Autodesk Inventor part; units mm, degrees
(part 2 of 2)
  arc A175 (-42.6526, 43.6661) -> (-42.977, 43.2779) centre (-40.6002, 41.6214) ccw
  line L41 (-42.977, 43.2779) -> (-43.1067, 43.0917)
  line L42 (-43.1067, 43.0917) -> (-41.872, 41.9259)
  line L43 (-41.872, 41.9259) -> (-40.6373, 40.7601)
  line L44 (-40.6373, 40.7601) -> (-40.3848, 41.0649)
  arc A176 (-39.3586, 42.1603) -> (-40.3848, 41.0649) centre (-30.9209, 33.2272) ccw
  arc A177 (-38.2304, 43.0935) -> (-39.3586, 42.1603) centre (-31.7148, 34.0677) ccw
  arc A178 (-37.0066, 43.858) -> (-38.2304, 43.0935) centre (-31.9087, 34.3364) ccw
  arc A179 (-35.6955, 44.45) -> (-37.0066, 43.858) centre (-31.97, 34.4509) ccw
  arc A180 (-32.3301, 45.1442) -> (-35.6955, 44.45) centre (-31.7654, 33.9017) ccw
  arc A181 (-28.9479, 44.7788) -> (-32.3301, 45.1442) centre (-31.7871, 34.3342) ccw
  arc A182 (-25.8331, 43.3785) -> (-28.9479, 44.7788) centre (-31.8114, 34.245) ccw
  arc A183 (-23.2452, 41.0656) -> (-25.8331, 43.3785) centre (-32.202, 33.6483) ccw
  line L45 (-23.2452, 41.0656) -> (-22.9934, 40.7615)
  line L46 (-22.9934, 40.7615) -> (-21.7595, 41.928)
  line L47 (-21.7595, 41.928) -> (-20.5256, 43.0945)
  line L48 (-20.5256, 43.0945) -> (-20.6545, 43.2793)
  arc A184 (-20.6545, 43.2793) -> (-20.7446, 43.3915) centre (-21.5367, 42.6637) ccw
  arc A185 (-20.7446, 43.3915) -> (-20.9906, 43.656) centre (-42.9217, 23.0143) ccw
  arc A186 (-20.9906, 43.656) -> (-21.2887, 43.9678) centre (-41.1575, 24.6748) ccw
  arc A187 (-21.2887, 43.9678) -> (-21.6175, 44.3024) centre (-49.0563, 17.0049) ccw
  arc A188 (-21.6175, 44.3024) -> (-22.5505, 45.1704) centre (-33.3143, 32.6659) ccw
  arc A189 (-22.5505, 45.1704) -> (-23.4953, 45.9106) centre (-31.0271, 35.323) ccw
  arc A190 (-23.4953, 45.9106) -> (-24.5028, 46.5592) centre (-31, 35.361) ccw
  arc A191 (-24.5028, 46.5592) -> (-25.6239, 47.1525) centre (-32.6544, 32.5096) ccw
  arc A192 (-25.6239, 47.1525) -> (-26.7379, 47.628) centre (-31.5598, 34.7894) ccw
  arc A193 (-26.7379, 47.628) -> (-27.9121, 48.0141) centre (-31.9655, 33.7091) ccw
  arc A194 (-27.9121, 48.0141) -> (-29.1159, 48.3018) centre (-31.976, 33.6721) ccw
  arc A195 (-29.1159, 48.3018) -> (-30.3185, 48.4827) centre (-31.7827, 34.6607) ccw
  arc A196 (-30.3185, 48.4827) -> (-30.9625, 48.5251) centre (-31.1728, 40.418) ccw
  arc A197 (-30.9625, 48.5251) -> (-31.8952, 48.5365) centre (-31.8434, 14.5791) ccw
  arc A198 (-31.8952, 48.5365) -> (-32.8196, 48.5227) centre (-31.8427, 14.0809) ccw
  arc A199 (-32.8196, 48.5227) -> (-33.4163, 48.478) centre (-32.6367, 42.0762) ccw
  arc A200 (-32.4307, 43.0264) -> (-34.0237, 42.7492) centre (-31.3613, 32.1655) ccw
  arc A201 (-34.0237, 42.7492) -> (-35.4688, 42.2479) centre (-31.8884, 34.261) ccw
  arc A202 (-35.4688, 42.2479) -> (-36.7759, 41.515) centre (-32.0428, 34.6053) ccw
  arc A203 (-36.7759, 41.515) -> (-37.9581, 40.5486) centre (-31.6765, 34.0706) ccw
  arc A204 (-37.9581, 40.5486) -> (-38.3376, 40.1652) centre (-28.7647, 31.0677) ccw
  arc A205 (-38.3376, 40.1652) -> (-38.6996, 39.7682) centre (-28.9248, 31.2199) ccw
  arc A206 (-38.6996, 39.7682) -> (-39.0151, 39.4003) centre (-20.0519, 23.4603) ccw
  arc A207 (-39.0151, 39.4003) -> (-39.0527, 39.2969) centre (-38.8921, 39.2969) ccw
  arc A208 (-39.0527, 39.2969) -> (-39.0335, 39.2524) centre (-38.9916, 39.2969) ccw
  arc A209 (-39.0335, 39.2524) -> (-37.8449, 38.1333) centre (2906.6809, 3166.558) ccw
  arc A210 (-37.8449, 38.1333) -> (-36.672, 37.0301) centre (1469.8323, 1639.9712) ccw
  arc A211 (-36.672, 37.0301) -> (-36.5889, 36.978) centre (-36.4978, 37.2154) ccw
  arc A212 (-36.5889, 36.978) -> (-36.5603, 36.9845) centre (-36.5795, 37.0026) ccw
  arc A213 (-36.5603, 36.9845) -> (-36.4741, 37.0791) centre (-39.0948, 39.3809) ccw
  arc A214 (-36.4741, 37.0791) -> (-36.3741, 37.2003) centre (-38.4073, 38.777) ccw
  arc A215 (-36.3741, 37.2003) -> (-36.2643, 37.3476) centre (-40.1553, 40.1326) ccw
  arc A216 (-35.6055, 38.1053) -> (-36.2643, 37.3476) centre (-31.9353, 34.249) ccw
  arc A217 (-34.8086, 38.7361) -> (-35.6055, 38.1053) centre (-31.7546, 34.0592) ccw
  arc A218 (-33.9056, 39.2153) -> (-34.8086, 38.7361) centre (-31.7182, 34.0034) ccw
  arc A219 (-32.9322, 39.5234) -> (-33.9056, 39.2153) centre (-31.7286, 34.0282) ccw
  arc A220 (-32.3612, 39.5988) -> (-32.9322, 39.5234) centre (-32.201, 36.1851) ccw
  arc A221 (-31.6217, 39.6035) -> (-32.3612, 39.5988) centre (-31.9333, 30.4803) ccw
  arc A222 (-30.8835, 39.5483) -> (-31.6217, 39.6035) centre (-31.9336, 30.4734) ccw
  arc A223 (-30.3166, 39.434) -> (-30.8835, 39.5483) centre (-31.2817, 36.1076) ccw
  arc A224 (-29.4512, 39.0947) -> (-30.3166, 39.434) centre (-31.7361, 34.5412) ccw
  arc A225 (-28.6193, 38.5905) -> (-29.4512, 39.0947) centre (-32.1874, 33.6419) ccw
  arc A226 (-27.8809, 37.9625) -> (-28.6193, 38.5905) centre (-32.1638, 33.6746) ccw
  arc A227 (-27.2937, 37.2545) -> (-27.8809, 37.9625) centre (-31.3579, 34.4814) ccw
  arc A228 (-27.2937, 37.2545) -> (-27.2128, 37.1424) centre (-25.1615, 38.7093) ccw
  arc A229 (-27.2128, 37.1424) -> (-27.1366, 37.051) centre (-26.0837, 38.0049) ccw
  arc A230 (-27.1366, 37.051) -> (-27.071, 36.9831) centre (-26.0649, 38.0219) ccw
  arc A231 (-27.071, 36.9831) -> (-27.0426, 36.9773) centre (-27.0522, 37.0025) ccw
  arc A232 (-27.0426, 36.9773) -> (-26.9623, 37.0275) centre (-27.13, 37.2061) ccw
  arc A233 (-26.9623, 37.0275) -> (-25.7864, 38.1315) centre (-1649.919, 1766.8952) ccw
  arc A234 (-25.7864, 38.1315) -> (-24.5953, 39.2509) centre (-3169.5689, 3384.4472) ccw
  arc A235 (-24.5953, 39.2509) -> (-24.5767, 39.2939) centre (-24.6358, 39.2939) ccw
  arc A236 (-24.5767, 39.2939) -> (-24.5825, 39.3115) centre (-24.6064, 39.2939) ccw
  arc A237 (-24.5825, 39.3115) -> (-24.6669, 39.4252) centre (-44.5732, 24.5671) ccw
  arc A238 (-24.6669, 39.4252) -> (-24.766, 39.5554) centre (-31.6067, 34.2453) ccw
  arc A239 (-24.766, 39.5554) -> (-24.8836, 39.7051) centre (-37.2564, 29.8598) ccw
  arc A240 (-24.8836, 39.7051) -> (-25.4949, 40.3815) centre (-30.5776, 35.1743) ccw
  arc A241 (-25.4949, 40.3815) -> (-26.2501, 41.0537) centre (-33.1647, 32.5237) ccw
  arc A242 (-26.2501, 41.0537) -> (-27.0662, 41.6552) centre (-33.1968, 32.4842) ccw
  arc A243 (-27.0662, 41.6552) -> (-27.8611, 42.1187) centre (-31.2352, 35.4187) ccw
  arc A244 (-27.8611, 42.1187) -> (-28.3727, 42.3447) centre (-30.3506, 37.1753) ccw
  arc A245 (-28.3727, 42.3447) -> (-29.0377, 42.5799) centre (-33.3146, 29.4285) ccw
  arc A246 (-29.0377, 42.5799) -> (-29.717, 42.7818) centre (-33.3337, 29.3697) ccw
  arc A247 (-29.717, 42.7818) -> (-30.2747, 42.9036) centre (-31.2556, 37.0763) ccw
  arc A248 (-30.2747, 42.9036) -> (-30.7758, 42.9692) centre (-31.4176, 36.1138) ccw
  arc A249 (-30.7758, 42.9692) -> (-31.4147, 43.0173) centre (-32.4141, 25.4701) ccw
  arc A250 (-31.4147, 43.0173) -> (-32.0314, 43.0416) centre (-32.4232, 25.3115) ccw
  arc A251 (-32.0314, 43.0416) -> (-32.4307, 43.0264) centre (-32.1049, 39.7171) ccw
  arc A252 (-32.5231, 37.4314) -> (-33.3556, 37.0457) centre (-31.7598, 34.6924) ccw
  arc A253 (-33.3556, 37.0457) -> (-34.029, 36.4127) centre (-31.7134, 34.624) ccw
  arc A254 (-34.029, 36.4127) -> (-34.4667, 35.6071) centre (-31.7526, 34.6543) ccw
  arc A255 (-34.4667, 35.6071) -> (-34.6168, 34.7211) centre (-31.9577, 34.7263) ccw
  arc A256 (-34.6168, 34.7211) -> (-34.3295, 33.4989) centre (-31.8505, 34.7265) ccw
  arc A257 (-34.3295, 33.4989) -> (-33.5302, 32.5168) centre (-31.7681, 34.7673) ccw
  arc A258 (-33.5302, 32.5168) -> (-32.39, 31.9809) centre (-31.7888, 34.7408) ccw
  arc A259 (-32.39, 31.9809) -> (-31.149, 32.0059) centre (-31.8219, 34.5891) ccw
  arc A260 (-31.149, 32.0059) -> (-30.4318, 32.2925) centre (-31.9281, 34.9968) ccw
  arc A261 (-30.4318, 32.2925) -> (-29.8377, 32.7398) centre (-31.7217, 34.6238) ccw
  arc A262 (-29.8377, 32.7398) -> (-29.3904, 33.3339) centre (-31.7217, 34.6238) ccw
  arc A263 (-29.3904, 33.3339) -> (-29.1038, 34.0512) centre (-32.0947, 34.8302) ccw
  arc A264 (-29.1038, 34.0512) -> (-29.0802, 35.3061) centre (-31.7012, 34.7277) ccw
  arc A265 (-29.0802, 35.3061) -> (-29.6276, 36.4511) centre (-31.8129, 34.703) ccw
  arc A266 (-29.6276, 36.4511) -> (-30.6294, 37.2438) centre (-31.8465, 34.6762) ccw
  arc A267 (-30.6294, 37.2438) -> (-31.8739, 37.5142) centre (-31.8323, 34.7062) ccw
  arc A268 (-31.8739, 37.5142) -> (-32.0366, 37.5064) centre (-31.837, 35.023) ccw
  arc A269 (-32.0366, 37.5064) -> (-32.2181, 37.4876) centre (-31.7229, 33.6029) ccw
  arc A270 (-32.2181, 37.4876) -> (-32.3905, 37.4614) centre (-31.75, 33.8157) ccw
  arc A271 (-32.3905, 37.4614) -> (-32.5231, 37.4314) centre (-32.15, 36.0926) ccw
  arc A272 (-54.2587, 71.8195) -> (-55.2164, 71.6633) centre (-53.721, 65.5053) ccw
  arc A273 (-55.2164, 71.6633) -> (-56.1281, 71.3638) centre (-53.7854, 65.7705) ccw
  arc A274 (-56.1281, 71.3638) -> (-56.9803, 70.9245) centre (-53.7898, 65.7811) ccw
  arc A275 (-56.9803, 70.9245) -> (-57.761, 70.3525) centre (-53.6689, 65.5862) ccw
  arc A276 (-57.761, 70.3525) -> (-57.9303, 70.1998) centre (-54.7143, 66.8038) ccw
  arc A277 (-57.9303, 70.1998) -> (-58.1244, 70.0106) centre (-51.5447, 63.4568) ccw
  arc A278 (-58.1244, 70.0106) -> (-58.3037, 69.8254) centre (-51.7023, 63.6139) ccw
  arc A279 (-58.3037, 69.8254) -> (-58.4189, 69.6921) centre (-56.7958, 68.4066) ccw
  line L49 (-58.4189, 69.6921) -> (-58.4764, 69.6194)
  line L50 (-58.4764, 69.6194) -> (-58.0951, 69.2684)
  line L51 (-58.0951, 69.2684) -> (-57.7138, 68.9174)
  line L52 (-57.7138, 68.9174) -> (-57.6118, 69.0338)
  arc A280 (-57.0139, 69.616) -> (-57.6118, 69.0338) centre (-53.6679, 65.5813) ccw
  arc A281 (-56.3308, 70.0963) -> (-57.0139, 69.616) centre (-53.6618, 65.5739) ccw
  arc A282 (-55.5869, 70.4582) -> (-56.3308, 70.0963) centre (-53.7111, 65.6576) ccw
  arc A283 (-54.8079, 70.6887) -> (-55.5869, 70.4582) centre (-53.8421, 65.9928) ccw
  arc A284 (-54.2943, 70.7669) -> (-54.8079, 70.6887) centre (-53.7974, 65.7752) ccw
  arc A285 (-53.7678, 70.793) -> (-54.2943, 70.7669) centre (-53.7678, 65.4777) ccw
  arc A286 (-53.2413, 70.7669) -> (-53.7678, 70.793) centre (-53.7678, 65.4777) ccw
  arc A287 (-52.7277, 70.6887) -> (-53.2413, 70.7669) centre (-53.7382, 65.7752) ccw
  arc A288 (-51.9486, 70.4585) -> (-52.7277, 70.6887) centre (-53.6976, 65.9726) ccw
  arc A289 (-51.2067, 70.0979) -> (-51.9486, 70.4585) centre (-53.8074, 65.6909) ccw
  arc A290 (-50.5247, 69.6182) -> (-51.2067, 70.0979) centre (-53.8645, 65.5942) ccw
  arc A291 (-49.9239, 69.034) -> (-50.5247, 69.6182) centre (-53.9323, 65.5125) ccw
  line L53 (-49.9239, 69.034) -> (-49.8218, 68.9178)
  line L54 (-49.8218, 68.9178) -> (-49.4403, 69.2684)
  line L55 (-49.4403, 69.2684) -> (-49.0588, 69.619)
  line L56 (-49.0588, 69.619) -> (-49.1187, 69.6961)
  arc A292 (-49.1187, 69.6961) -> (-49.2435, 69.8387) centre (-50.3783, 68.7188) ccw
  arc A293 (-49.2435, 69.8387) -> (-49.4908, 70.0838) centre (-60.4502, 58.7794) ccw
  arc A294 (-49.4908, 70.0838) -> (-49.7488, 70.3278) centre (-59.4752, 59.7852) ccw
  arc A295 (-49.7488, 70.3278) -> (-49.9351, 70.4876) centre (-52.0641, 67.8182) ccw
  arc A296 (-49.9351, 70.4876) -> (-50.698, 71.0097) centre (-53.8793, 65.5422) ccw
  arc A297 (-50.698, 71.0097) -> (-51.5212, 71.4089) centre (-53.7491, 65.766) ccw
  arc A298 (-51.5212, 71.4089) -> (-52.3959, 71.6801) centre (-53.7544, 65.7527) ccw
  arc A299 (-52.3959, 71.6801) -> (-53.3127, 71.8212) centre (-53.8245, 65.4466) ccw
  arc A300 (-53.3127, 71.8212) -> (-53.5357, 71.8337) centre (-53.6841, 67.195) ccw
  arc A301 (-53.5357, 71.8337) -> (-53.7872, 71.8375) centre (-53.7737, 64.3958) ccw
  arc A302 (-53.7872, 71.8375) -> (-54.0379, 71.8328) centre (-53.7737, 64.4287) ccw
  arc A303 (-54.0379, 71.8328) -> (-54.2587, 71.8195) centre (-53.8779, 67.3479) ccw
  arc A304 (-54.2587, 70.1206) -> (-54.8466, 70.011) centre (-53.685, 65.4098) ccw
  arc A305 (-54.8466, 70.011) -> (-55.4044, 69.8298) centre (-53.7721, 65.755) ccw
  arc A306 (-55.4044, 69.8298) -> (-55.9344, 69.5753) centre (-53.7639, 65.7344) ccw
  arc A307 (-55.9344, 69.5753) -> (-56.4394, 69.2471) centre (-53.5452, 65.3475) ccw
  arc A308 (-56.4394, 69.2471) -> (-56.6021, 69.1131) centre (-55.1906, 67.5645) ccw
  arc A309 (-56.6021, 69.1131) -> (-56.8494, 68.8817) centre (-47.9272, 59.5958) ccw
  arc A310 (-56.8494, 68.8817) -> (-57.0896, 68.6458) centre (-46.1793, 57.7765) ccw
  arc A311 (-57.0896, 68.6458) -> (-57.189, 68.5268) centre (-56.4605, 68.0191) ccw
  line L57 (-57.189, 68.5268) -> (-57.2288, 68.4697)
  line L58 (-57.2288, 68.4697) -> (-56.8503, 68.1124)
  line L59 (-56.8503, 68.1124) -> (-56.4719, 67.7551)
  line L60 (-56.4719, 67.7551) -> (-56.3945, 67.8485)
  arc A312 (-56.08, 68.1842) -> (-56.3945, 67.8485) centre (-53.4938, 65.4462) ccw
  arc A313 (-55.7342, 68.4703) -> (-56.08, 68.1842) centre (-53.7371, 65.7039) ccw
  arc A314 (-55.3591, 68.7046) -> (-55.7342, 68.4703) centre (-53.7966, 65.7862) ccw
  arc A315 (-54.9572, 68.886) -> (-55.3591, 68.7046) centre (-53.8154, 65.8213) ccw
  arc A316 (-53.9257, 69.0988) -> (-54.9572, 68.886) centre (-53.7527, 65.653) ccw
  arc A317 (-52.8891, 68.9868) -> (-53.9257, 69.0988) centre (-53.7593, 65.7856) ccw
  arc A318 (-51.9344, 68.5576) -> (-52.8891, 68.9868) centre (-53.7667, 65.7582) ccw
  arc A319 (-51.1412, 67.8487) -> (-51.9344, 68.5576) centre (-53.8865, 65.5753) ccw
  line L61 (-51.1412, 67.8487) -> (-51.064, 67.7555)
  line L62 (-51.064, 67.7555) -> (-50.6858, 68.113)
  line L63 (-50.6858, 68.113) -> (-50.3077, 68.4706)
  line L64 (-50.3077, 68.4706) -> (-50.3472, 68.5272)
  arc A320 (-50.3472, 68.5272) -> (-50.3748, 68.5616) centre (-50.6176, 68.3385) ccw
  arc A321 (-50.3748, 68.5616) -> (-50.4502, 68.6427) centre (-57.1721, 62.316) ccw
  arc A322 (-50.4502, 68.6427) -> (-50.5416, 68.7383) centre (-56.6313, 62.825) ccw
  arc A323 (-50.5416, 68.7383) -> (-50.6423, 68.8408) centre (-59.0523, 60.4741) ccw
  arc A324 (-50.6423, 68.8408) -> (-50.9283, 69.1069) centre (-54.2274, 65.2742) ccw
  arc A325 (-50.9283, 69.1069) -> (-51.2179, 69.3337) centre (-53.5264, 66.0886) ccw
  arc A326 (-51.2179, 69.3337) -> (-51.5267, 69.5325) centre (-53.5181, 66.1003) ccw
  arc A327 (-51.5267, 69.5325) -> (-51.8703, 69.7143) centre (-54.0251, 65.2263) ccw
  arc A328 (-51.8703, 69.7143) -> (-52.2117, 69.8601) centre (-53.6897, 65.9251) ccw
  arc A329 (-52.2117, 69.8601) -> (-52.5716, 69.9784) centre (-53.814, 65.594) ccw
  arc A330 (-52.5716, 69.9784) -> (-52.9406, 70.0666) centre (-53.8172, 65.5826) ccw
  arc A331 (-52.9406, 70.0666) -> (-53.3092, 70.1221) centre (-53.758, 65.8856) ccw
  arc A332 (-53.3092, 70.1221) -> (-53.5066, 70.1351) centre (-53.571, 67.6502) ccw
  arc A333 (-53.5066, 70.1351) -> (-53.7925, 70.1386) centre (-53.7766, 59.7306) ccw
  arc A334 (-53.7925, 70.1386) -> (-54.0758, 70.1343) centre (-53.7763, 59.5779) ccw
  arc A335 (-54.0758, 70.1343) -> (-54.2587, 70.1206) centre (-54.0197, 68.1585) ccw
  arc A336 (-53.9566, 68.4497) -> (-54.4448, 68.3648) centre (-53.6288, 65.1208) ccw
  arc A337 (-54.4448, 68.3648) -> (-54.8878, 68.2111) centre (-53.7904, 65.7631) ccw
  arc A338 (-54.8878, 68.2111) -> (-55.2884, 67.9865) centre (-53.8377, 65.8687) ccw
  arc A339 (-55.2884, 67.9865) -> (-55.6507, 67.6903) centre (-53.7254, 65.7048) ccw
  arc A340 (-55.6507, 67.6903) -> (-55.7671, 67.5728) centre (-52.8329, 64.7844) ccw
  arc A341 (-55.7671, 67.5728) -> (-55.878, 67.4511) centre (-52.882, 64.831) ccw
  arc A342 (-55.878, 67.4511) -> (-55.9747, 67.3383) centre (-50.1625, 62.4527) ccw
  arc A343 (-55.9747, 67.3383) -> (-55.9862, 67.3066) centre (-55.937, 67.3066) ccw
  arc A344 (-55.9862, 67.3066) -> (-55.9803, 67.293) centre (-55.9675, 67.3066) ccw
  arc A345 (-55.9803, 67.293) -> (-55.616, 66.95) centre (846.8811, 1025.8121) ccw
  arc A346 (-55.616, 66.95) -> (-55.2565, 66.6118) centre (406.487, 557.9133) ccw
  arc A347 (-55.2565, 66.6118) -> (-55.2311, 66.5959) centre (-55.2031, 66.6687) ccw
  arc A348 (-55.2311, 66.5959) -> (-55.2223, 66.5979) centre (-55.2282, 66.6034) ccw
  arc A349 (-55.2223, 66.5979) -> (-55.1959, 66.6269) centre (-55.9991, 67.3324) ccw
  arc A350 (-55.1959, 66.6269) -> (-55.1652, 66.664) centre (-55.7884, 67.1473) ccw
  arc A351 (-55.1652, 66.664) -> (-55.1316, 66.7092) centre (-56.3242, 67.5628) ccw
  arc A352 (-54.9296, 66.9414) -> (-55.1316, 66.7092) centre (-53.8047, 65.7595) ccw
  arc A353 (-54.6854, 67.1347) -> (-54.9296, 66.9414) centre (-53.7494, 65.7013) ccw
  arc A354 (-54.4086, 67.2816) -> (-54.6854, 67.1347) centre (-53.7382, 65.6842) ccw
  arc A355 (-54.1103, 67.376) -> (-54.4086, 67.2816) centre (-53.7414, 65.6918) ccw
  arc A356 (-53.9353, 67.3991) -> (-54.1103, 67.376) centre (-53.8862, 66.3529) ccw
  arc A357 (-53.7086, 67.4006) -> (-53.9353, 67.3991) centre (-53.8041, 64.6043) ccw
  arc A358 (-53.4824, 67.3837) -> (-53.7086, 67.4006) centre (-53.8042, 64.6022) ccw
  arc A359 (-53.3086, 67.3487) -> (-53.4824, 67.3837) centre (-53.6044, 66.3291) ccw
  arc A360 (-53.0433, 67.2446) -> (-53.3086, 67.3487) centre (-53.7437, 65.849) ccw
  arc A361 (-52.7884, 67.0901) -> (-53.0433, 67.2446) centre (-53.882, 65.5734) ccw
  arc A362 (-52.562, 66.8976) -> (-52.7884, 67.0901) centre (-53.8748, 65.5834) ccw
  arc A363 (-52.3821, 66.6806) -> (-52.562, 66.8976) centre (-53.6278, 65.8307) ccw
  arc A364 (-52.3821, 66.6806) -> (-52.3573, 66.6463) centre (-51.7286, 67.1265) ccw
  arc A365 (-52.3573, 66.6463) -> (-52.3339, 66.6182) centre (-52.0112, 66.9106) ccw
  arc A366 (-52.3339, 66.6182) -> (-52.3138, 66.5974) centre (-52.0055, 66.9158) ccw
  arc A367 (-52.3138, 66.5974) -> (-52.3051, 66.5957) centre (-52.3081, 66.6034) ccw
  arc A368 (-52.3051, 66.5957) -> (-52.2805, 66.611) centre (-52.3319, 66.6658) ccw
  arc A369 (-52.2805, 66.611) -> (-51.9201, 66.9494) centre (-549.7167, 596.8155) ccw
  arc A370 (-51.9201, 66.9494) -> (-51.555, 67.2925) centre (-1015.4894, 1092.5952) ccw
  arc A371 (-51.555, 67.2925) -> (-51.5493, 67.3057) centre (-51.5674, 67.3057) ccw
  arc A372 (-51.5493, 67.3057) -> (-51.5511, 67.3111) centre (-51.5584, 67.3057) ccw
  arc A373 (-51.5511, 67.3111) -> (-51.577, 67.3459) centre (-57.6783, 62.7919) ccw
  arc A374 (-51.577, 67.3459) -> (-51.6073, 67.3859) centre (-53.704, 65.7583) ccw
  arc A375 (-51.6073, 67.3859) -> (-51.6434, 67.4317) centre (-55.4356, 64.4141) ccw
  arc A376 (-51.6434, 67.4317) -> (-51.8307, 67.6391) centre (-53.3886, 66.043) ccw
  arc A377 (-51.8307, 67.6391) -> (-52.0622, 67.8451) centre (-54.1816, 65.2306) ccw
  arc A378 (-52.0622, 67.8451) -> (-52.3124, 68.0294) centre (-54.1914, 65.2185) ccw
  arc A379 (-52.3124, 68.0294) -> (-52.556, 68.1715) centre (-53.5902, 66.1179) ccw
  arc A380 (-52.556, 68.1715) -> (-52.7128, 68.2408) centre (-53.319, 66.6563) ccw
  arc A381 (-52.7128, 68.2408) -> (-52.9166, 68.3129) centre (-54.2275, 64.282) ccw
  arc A382 (-52.9166, 68.3129) -> (-53.1248, 68.3747) centre (-54.2334, 64.2639) ccw
  arc A383 (-53.1248, 68.3747) -> (-53.2958, 68.4121) centre (-53.5964, 66.626) ccw
  arc A384 (-53.2958, 68.4121) -> (-53.4493, 68.4322) centre (-53.6461, 66.331) ccw
  arc A385 (-53.4493, 68.4322) -> (-53.6452, 68.4469) centre (-53.9515, 63.0687) ccw
  arc A386 (-53.6452, 68.4469) -> (-53.8342, 68.4544) centre (-53.9543, 63.0201) ccw
  arc A387 (-53.8342, 68.4544) -> (-53.9566, 68.4497) centre (-53.8567, 67.4354) ccw
  arc A388 (-53.9849, 66.7348) -> (-54.24, 66.6166) centre (-53.7509, 65.8954) ccw
  arc A389 (-54.24, 66.6166) -> (-54.4464, 66.4226) centre (-53.7367, 65.8744) ccw
  arc A390 (-54.4464, 66.4226) -> (-54.5806, 66.1757) centre (-53.7487, 65.8837) ccw
  arc A391 (-54.5806, 66.1757) -> (-54.6266, 65.9041) centre (-53.8116, 65.9057) ccw
  arc A392 (-54.6266, 65.9041) -> (-54.5386, 65.5295) centre (-53.7788, 65.9058) ccw
  arc A393 (-54.5386, 65.5295) -> (-54.2936, 65.2285) centre (-53.7535, 65.9183) ccw
  arc A394 (-54.2936, 65.2285) -> (-53.9441, 65.0643) centre (-53.7598, 65.9102) ccw
  arc A395 (-53.9441, 65.0643) -> (-53.5637, 65.0719) centre (-53.77, 65.8637) ccw
  arc A396 (-53.5637, 65.0719) -> (-53.3439, 65.1598) centre (-53.8025, 65.9887) ccw
  arc A397 (-53.3439, 65.1598) -> (-53.1618, 65.2969) centre (-53.7393, 65.8743) ccw
  arc A398 (-53.1618, 65.2969) -> (-53.0247, 65.479) centre (-53.7393, 65.8743) ccw
  arc A399 (-53.0247, 65.479) -> (-52.9369, 65.6988) centre (-53.8536, 65.9376) ccw
  arc A400 (-52.9369, 65.6988) -> (-52.9297, 66.0834) centre (-53.733, 65.9062) ccw
  arc A401 (-52.9297, 66.0834) -> (-53.0974, 66.4344) centre (-53.7672, 65.8986) ccw
  arc A402 (-53.0974, 66.4344) -> (-53.4045, 66.6773) centre (-53.7775, 65.8904) ccw
  arc A403 (-53.4045, 66.6773) -> (-53.7859, 66.7602) centre (-53.7732, 65.8996) ccw
  arc A404 (-53.7859, 66.7602) -> (-53.8358, 66.7578) centre (-53.7746, 65.9967) ccw
  arc A405 (-53.8358, 66.7578) -> (-53.8914, 66.7521) centre (-53.7396, 65.5614) ccw
  arc A406 (-53.8914, 66.7521) -> (-53.9443, 66.7441) centre (-53.7479, 65.6266) ccw
  arc A407 (-53.9443, 66.7441) -> (-53.9849, 66.7348) centre (-53.8705, 66.3245) ccw
  arc A408 (-9.2413, 17.0805) -> (-8.2836, 17.2367) centre (-9.779, 23.3947) ccw
  arc A409 (-8.2836, 17.2367) -> (-7.3719, 17.5362) centre (-9.7146, 23.1295) ccw
  arc A410 (-7.3719, 17.5362) -> (-6.5197, 17.9755) centre (-9.7102, 23.1189) ccw
  arc A411 (-6.5197, 17.9755) -> (-5.739, 18.5475) centre (-9.8311, 23.3138) ccw
  arc A412 (-5.739, 18.5475) -> (-5.5697, 18.7002) centre (-8.7857, 22.0962) ccw
  arc A413 (-5.5697, 18.7002) -> (-5.3756, 18.8894) centre (-11.9553, 25.4432) ccw
  arc A414 (-5.3756, 18.8894) -> (-5.1963, 19.0746) centre (-11.7977, 25.2861) ccw
  arc A415 (-5.1963, 19.0746) -> (-5.0811, 19.2079) centre (-6.7042, 20.4934) ccw
  line L65 (-5.0811, 19.2079) -> (-5.0236, 19.2806)
  line L66 (-5.0236, 19.2806) -> (-5.4049, 19.6316)
  line L67 (-5.4049, 19.6316) -> (-5.7862, 19.9826)
  line L68 (-5.7862, 19.9826) -> (-5.8882, 19.8662)
  arc A416 (-6.4861, 19.284) -> (-5.8882, 19.8662) centre (-9.8321, 23.3187) ccw
  arc A417 (-7.1692, 18.8037) -> (-6.4861, 19.284) centre (-9.8382, 23.3261) ccw
  arc A418 (-7.9131, 18.4418) -> (-7.1692, 18.8037) centre (-9.7889, 23.2424) ccw
  arc A419 (-8.6921, 18.2113) -> (-7.9131, 18.4418) centre (-9.6579, 22.9072) ccw
  arc A420 (-9.2057, 18.1331) -> (-8.6921, 18.2113) centre (-9.7026, 23.1248) ccw
  arc A421 (-9.7322, 18.107) -> (-9.2057, 18.1331) centre (-9.7322, 23.4223) ccw
  arc A422 (-10.2587, 18.1331) -> (-9.7322, 18.107) centre (-9.7322, 23.4223) ccw
  arc A423 (-10.7723, 18.2113) -> (-10.2587, 18.1331) centre (-9.7618, 23.1248) ccw
  arc A424 (-11.5514, 18.4415) -> (-10.7723, 18.2113) centre (-9.8024, 22.9274) ccw
  arc A425 (-12.2933, 18.8021) -> (-11.5514, 18.4415) centre (-9.6926, 23.2091) ccw
  arc A426 (-12.9753, 19.2818) -> (-12.2933, 18.8021) centre (-9.6355, 23.3058) ccw
  arc A427 (-13.5761, 19.866) -> (-12.9753, 19.2818) centre (-9.5677, 23.3875) ccw
  line L69 (-13.5761, 19.866) -> (-13.6782, 19.9822)
  line L70 (-13.6782, 19.9822) -> (-14.0597, 19.6316)
  line L71 (-14.0597, 19.6316) -> (-14.4412, 19.281)
  line L72 (-14.4412, 19.281) -> (-14.3813, 19.2039)
  arc A428 (-14.3813, 19.2039) -> (-14.2565, 19.0613) centre (-13.1217, 20.1812) ccw
  arc A429 (-14.2565, 19.0613) -> (-14.0092, 18.8162) centre (-3.0498, 30.1206) ccw
  arc A430 (-14.0092, 18.8162) -> (-13.7512, 18.5722) centre (-4.0248, 29.1148) ccw
  arc A431 (-13.7512, 18.5722) -> (-13.5649, 18.4124) centre (-11.4359, 21.0818) ccw
  arc A432 (-13.5649, 18.4124) -> (-12.802, 17.8903) centre (-9.6207, 23.3578) ccw
  arc A433 (-12.802, 17.8903) -> (-11.9788, 17.4911) centre (-9.7509, 23.134) ccw
  arc A434 (-11.9788, 17.4911) -> (-11.1041, 17.2199) centre (-9.7456, 23.1473) ccw
  arc A435 (-11.1041, 17.2199) -> (-10.1873, 17.0788) centre (-9.6755, 23.4534) ccw
  arc A436 (-10.1873, 17.0788) -> (-9.9643, 17.0663) centre (-9.8159, 21.705) ccw
  arc A437 (-9.9643, 17.0663) -> (-9.7128, 17.0625) centre (-9.7263, 24.5042) ccw
  arc A438 (-9.7128, 17.0625) -> (-9.4621, 17.0672) centre (-9.7263, 24.4713) ccw
  arc A439 (-9.4621, 17.0672) -> (-9.2413, 17.0805) centre (-9.6221, 21.5521) ccw
  arc A440 (-9.2413, 18.7794) -> (-8.6534, 18.889) centre (-9.815, 23.4902) ccw
  arc A441 (-8.6534, 18.889) -> (-8.0956, 19.0702) centre (-9.7279, 23.145) ccw
  arc A442 (-8.0956, 19.0702) -> (-7.5656, 19.3247) centre (-9.7361, 23.1656) ccw
  arc A443 (-7.5656, 19.3247) -> (-7.0606, 19.6529) centre (-9.9548, 23.5525) ccw
  arc A444 (-7.0606, 19.6529) -> (-6.8979, 19.7869) centre (-8.3094, 21.3355) ccw
  arc A445 (-6.8979, 19.7869) -> (-6.6506, 20.0183) centre (-15.5728, 29.3042) ccw
  arc A446 (-6.6506, 20.0183) -> (-6.4104, 20.2542) centre (-17.3207, 31.1235) ccw
  arc A447 (-6.4104, 20.2542) -> (-6.311, 20.3732) centre (-7.0395, 20.8809) ccw
  line L73 (-6.311, 20.3732) -> (-6.2712, 20.4303)
  line L74 (-6.2712, 20.4303) -> (-6.6497, 20.7876)
  line L75 (-6.6497, 20.7876) -> (-7.0281, 21.1449)
  line L76 (-7.0281, 21.1449) -> (-7.1055, 21.0515)
  arc A448 (-7.42, 20.7158) -> (-7.1055, 21.0515) centre (-10.0062, 23.4538) ccw
  arc A449 (-7.7658, 20.4297) -> (-7.42, 20.7158) centre (-9.7629, 23.1961) ccw
  arc A450 (-8.1409, 20.1954) -> (-7.7658, 20.4297) centre (-9.7034, 23.1138) ccw
  arc A451 (-8.5428, 20.014) -> (-8.1409, 20.1954) centre (-9.6846, 23.0787) ccw
  arc A452 (-9.5743, 19.8012) -> (-8.5428, 20.014) centre (-9.7473, 23.247) ccw
  arc A453 (-10.6109, 19.9132) -> (-9.5743, 19.8012) centre (-9.7407, 23.1144) ccw
  arc A454 (-11.5656, 20.3424) -> (-10.6109, 19.9132) centre (-9.7333, 23.1418) ccw
  arc A455 (-12.3588, 21.0513) -> (-11.5656, 20.3424) centre (-9.6135, 23.3247) ccw
  line L77 (-12.3588, 21.0513) -> (-12.436, 21.1445)
  line L78 (-12.436, 21.1445) -> (-12.8142, 20.787)
  line L79 (-12.8142, 20.787) -> (-13.1923, 20.4294)
  line L80 (-13.1923, 20.4294) -> (-13.1528, 20.3728)
  arc A456 (-13.1528, 20.3728) -> (-13.1252, 20.3384) centre (-12.8824, 20.5615) ccw
  arc A457 (-13.1252, 20.3384) -> (-13.0498, 20.2573) centre (-6.3279, 26.584) ccw
  arc A458 (-13.0498, 20.2573) -> (-12.9584, 20.1617) centre (-6.8687, 26.075) ccw
  arc A459 (-12.9584, 20.1617) -> (-12.8577, 20.0592) centre (-4.4477, 28.4259) ccw
  arc A460 (-12.8577, 20.0592) -> (-12.5717, 19.7931) centre (-9.2726, 23.6258) ccw
  arc A461 (-12.5717, 19.7931) -> (-12.2821, 19.5663) centre (-9.9736, 22.8114) ccw
  arc A462 (-12.2821, 19.5663) -> (-11.9733, 19.3675) centre (-9.9819, 22.7997) ccw
  arc A463 (-11.9733, 19.3675) -> (-11.6297, 19.1857) centre (-9.4749, 23.6737) ccw
  arc A464 (-11.6297, 19.1857) -> (-11.2883, 19.0399) centre (-9.8103, 22.9749) ccw
  arc A465 (-11.2883, 19.0399) -> (-10.9284, 18.9216) centre (-9.686, 23.306) ccw
  arc A466 (-10.9284, 18.9216) -> (-10.5594, 18.8334) centre (-9.6828, 23.3174) ccw
  arc A467 (-10.5594, 18.8334) -> (-10.1908, 18.7779) centre (-9.742, 23.0144) ccw
  arc A468 (-10.1908, 18.7779) -> (-9.9934, 18.7649) centre (-9.929, 21.2498) ccw
  arc A469 (-9.9934, 18.7649) -> (-9.7075, 18.7614) centre (-9.7234, 29.1694) ccw
  arc A470 (-9.7075, 18.7614) -> (-9.4242, 18.7657) centre (-9.7237, 29.3221) ccw
  arc A471 (-9.4242, 18.7657) -> (-9.2413, 18.7794) centre (-9.4803, 20.7415) ccw
  arc A472 (-9.5434, 20.4503) -> (-9.0552, 20.5352) centre (-9.8712, 23.7792) ccw
  arc A473 (-9.0552, 20.5352) -> (-8.6122, 20.6889) centre (-9.7096, 23.1369) ccw
  arc A474 (-8.6122, 20.6889) -> (-8.2116, 20.9135) centre (-9.6623, 23.0313) ccw
  arc A475 (-8.2116, 20.9135) -> (-7.8493, 21.2097) centre (-9.7746, 23.1952) ccw
  arc A476 (-7.8493, 21.2097) -> (-7.7329, 21.3272) centre (-10.6671, 24.1156) ccw
  arc A477 (-7.7329, 21.3272) -> (-7.622, 21.4489) centre (-10.618, 24.069) ccw
  arc A478 (-7.622, 21.4489) -> (-7.5253, 21.5617) centre (-13.3375, 26.4473) ccw
  arc A479 (-7.5253, 21.5617) -> (-7.5138, 21.5934) centre (-7.563, 21.5934) ccw
  arc A480 (-7.5138, 21.5934) -> (-7.5197, 21.607) centre (-7.5325, 21.5934) ccw
  arc A481 (-7.5197, 21.607) -> (-7.884, 21.95) centre (-910.3811, -936.9121) ccw
  arc A482 (-7.884, 21.95) -> (-8.2435, 22.2882) centre (-469.987, -469.0133) ccw
  arc A483 (-8.2435, 22.2882) -> (-8.2689, 22.3041) centre (-8.2969, 22.2313) ccw
  arc A484 (-8.2689, 22.3041) -> (-8.2777, 22.3021) centre (-8.2718, 22.2966) ccw
  arc A485 (-8.2777, 22.3021) -> (-8.3041, 22.2731) centre (-7.5009, 21.5676) ccw
  arc A486 (-8.3041, 22.2731) -> (-8.3348, 22.236) centre (-7.7116, 21.7527) ccw
  arc A487 (-8.3348, 22.236) -> (-8.3684, 22.1908) centre (-7.1758, 21.3372) ccw
  arc A488 (-8.5704, 21.9586) -> (-8.3684, 22.1908) centre (-9.6953, 23.1405) ccw
  arc A489 (-8.8146, 21.7653) -> (-8.5704, 21.9586) centre (-9.7506, 23.1987) ccw
  arc A490 (-9.0914, 21.6184) -> (-8.8146, 21.7653) centre (-9.7618, 23.2158) ccw
  arc A491 (-9.3897, 21.524) -> (-9.0914, 21.6184) centre (-9.7586, 23.2082) ccw
  arc A492 (-9.5647, 21.5009) -> (-9.3897, 21.524) centre (-9.6138, 22.5471) ccw
  arc A493 (-9.7914, 21.4994) -> (-9.5647, 21.5009) centre (-9.6959, 24.2957) ccw
  arc A494 (-10.0176, 21.5163) -> (-9.7914, 21.4994) centre (-9.6958, 24.2978) ccw
  arc A495 (-10.1914, 21.5513) -> (-10.0176, 21.5163) centre (-9.8956, 22.5709) ccw
  arc A496 (-10.4567, 21.6554) -> (-10.1914, 21.5513) centre (-9.7563, 23.051) ccw
  arc A497 (-10.7116, 21.8099) -> (-10.4567, 21.6554) centre (-9.618, 23.3266) ccw
  arc A498 (-10.938, 22.0024) -> (-10.7116, 21.8099) centre (-9.6252, 23.3166) ccw
  arc A499 (-11.1179, 22.2194) -> (-10.938, 22.0024) centre (-9.8722, 23.0693) ccw
  arc A500 (-11.1179, 22.2194) -> (-11.1427, 22.2537) centre (-11.7714, 21.7735) ccw
  arc A501 (-11.1427, 22.2537) -> (-11.1661, 22.2818) centre (-11.4888, 21.9894) ccw
  arc A502 (-11.1661, 22.2818) -> (-11.1862, 22.3026) centre (-11.4945, 21.9842) ccw
  arc A503 (-11.1862, 22.3026) -> (-11.1949, 22.3043) centre (-11.1919, 22.2966) ccw
  arc A504 (-11.1949, 22.3043) -> (-11.2195, 22.289) centre (-11.1681, 22.2342) ccw
  arc A505 (-11.2195, 22.289) -> (-11.5799, 21.9506) centre (486.2167, -507.9155) ccw
  arc A506 (-11.5799, 21.9506) -> (-11.945, 21.6075) centre (951.9894, -1003.6952) ccw
  arc A507 (-11.945, 21.6075) -> (-11.9507, 21.5943) centre (-11.9326, 21.5943) ccw
  arc A508 (-11.9507, 21.5943) -> (-11.9489, 21.5889) centre (-11.9416, 21.5943) ccw
  arc A509 (-11.9489, 21.5889) -> (-11.923, 21.5541) centre (-5.8217, 26.1081) ccw
  arc A510 (-11.923, 21.5541) -> (-11.8927, 21.5141) centre (-9.796, 23.1417) ccw
  arc A511 (-11.8927, 21.5141) -> (-11.8566, 21.4683) centre (-8.0644, 24.4859) ccw
  arc A512 (-11.8566, 21.4683) -> (-11.6693, 21.2609) centre (-10.1114, 22.857) ccw
  arc A513 (-11.6693, 21.2609) -> (-11.4378, 21.0549) centre (-9.3184, 23.6694) ccw
  arc A514 (-11.4378, 21.0549) -> (-11.1876, 20.8706) centre (-9.3086, 23.6815) ccw
  arc A515 (-11.1876, 20.8706) -> (-10.944, 20.7285) centre (-9.9098, 22.7821) ccw
  arc A516 (-10.944, 20.7285) -> (-10.7872, 20.6592) centre (-10.181, 22.2437) ccw
  arc A517 (-10.7872, 20.6592) -> (-10.5834, 20.5871) centre (-9.2725, 24.618) ccw
  arc A518 (-10.5834, 20.5871) -> (-10.3752, 20.5253) centre (-9.2666, 24.6361) ccw
  arc A519 (-10.3752, 20.5253) -> (-10.2042, 20.4879) centre (-9.9036, 22.274) ccw
  arc A520 (-10.2042, 20.4879) -> (-10.0507, 20.4678) centre (-9.8539, 22.569) ccw
  arc A521 (-10.0507, 20.4678) -> (-9.8548, 20.4531) centre (-9.5485, 25.8313) ccw
  arc A522 (-9.8548, 20.4531) -> (-9.6658, 20.4456) centre (-9.5457, 25.8799) ccw
  arc A523 (-9.6658, 20.4456) -> (-9.5434, 20.4503) centre (-9.6433, 21.4646) ccw
  arc A524 (-9.5151, 22.1652) -> (-9.26, 22.2834) centre (-9.7491, 23.0046) ccw
  arc A525 (-9.26, 22.2834) -> (-9.0536, 22.4774) centre (-9.7633, 23.0256) ccw
  arc A526 (-9.0536, 22.4774) -> (-8.9194, 22.7243) centre (-9.7513, 23.0163) ccw
  arc A527 (-8.9194, 22.7243) -> (-8.8734, 22.9959) centre (-9.6884, 22.9943) ccw
  arc A528 (-8.8734, 22.9959) -> (-8.9614, 23.3705) centre (-9.7212, 22.9942) ccw
  arc A529 (-8.9614, 23.3705) -> (-9.2064, 23.6715) centre (-9.7465, 22.9817) ccw
  arc A530 (-9.2064, 23.6715) -> (-9.5559, 23.8357) centre (-9.7402, 22.9898) ccw
  arc A531 (-9.5559, 23.8357) -> (-9.9363, 23.8281) centre (-9.73, 23.0363) ccw
  arc A532 (-9.9363, 23.8281) -> (-10.1561, 23.7402) centre (-9.6975, 22.9113) ccw
  arc A533 (-10.1561, 23.7402) -> (-10.3382, 23.6031) centre (-9.7607, 23.0257) ccw
  arc A534 (-10.3382, 23.6031) -> (-10.4753, 23.421) centre (-9.7607, 23.0257) ccw
  arc A535 (-10.4753, 23.421) -> (-10.5631, 23.2012) centre (-9.6464, 22.9624) ccw
  arc A536 (-10.5631, 23.2012) -> (-10.5703, 22.8166) centre (-9.767, 22.9938) ccw
  arc A537 (-10.5703, 22.8166) -> (-10.4026, 22.4656) centre (-9.7328, 23.0014) ccw
  arc A538 (-10.4026, 22.4656) -> (-10.0955, 22.2227) centre (-9.7225, 23.0096) ccw
  arc A539 (-10.0955, 22.2227) -> (-9.7141, 22.1398) centre (-9.7268, 23.0004) ccw
  arc A540 (-9.7141, 22.1398) -> (-9.6642, 22.1422) centre (-9.7254, 22.9033) ccw
  arc A541 (-9.6642, 22.1422) -> (-9.6086, 22.1479) centre (-9.7604, 23.3386) ccw
  arc A542 (-9.6086, 22.1479) -> (-9.5557, 22.1559) centre (-9.7521, 23.2734) ccw
  arc A543 (-9.5557, 22.1559) -> (-9.5151, 22.1652) centre (-9.6295, 22.5755) ccw
  line L81 (-58.0705, 75.4711) -> (-54.6454, 85.6311)
  line L82 (-54.6454, 85.6311) -> (-52.9822, 85.6311)
  line L83 (-52.9822, 85.6311) -> (-49.5571, 75.4711)
  line L84 (-49.5571, 75.4711) -> (-50.9815, 75.4711)
  line L85 (-50.9815, 75.4711) -> (-51.9037, 78.3116)
  line L86 (-51.9037, 78.3116) -> (-55.7816, 78.3116)
  line L87 (-55.7816, 78.3116) -> (-56.7037, 75.4711)
  line L88 (-56.7037, 75.4711) -> (-58.0705, 75.4711)
  line L89 (-52.2742, 79.4643) -> (-53.8467, 84.2479)
  line L90 (-53.8467, 84.2479) -> (-55.4111, 79.4643)
  line L91 (-55.4111, 79.4643) -> (-52.2742, 79.4643)
  line L92 (-5.4295, 13.7735) -> (-8.8546, 3.6135)
  line L93 (-8.8546, 3.6135) -> (-10.5178, 3.6135)
  line L94 (-10.5178, 3.6135) -> (-13.9429, 13.7735)
  line L95 (-13.9429, 13.7735) -> (-12.5185, 13.7735)
  line L96 (-12.5185, 13.7735) -> (-11.5963, 10.9329)
  line L97 (-11.5963, 10.9329) -> (-7.7184, 10.9329)
  line L98 (-7.7184, 10.9329) -> (-6.7963, 13.7735)
  line L99 (-6.7963, 13.7735) -> (-5.4295, 13.7735)
  line L100 (-11.2258, 9.7803) -> (-9.6533, 4.9967)
  line L101 (-9.6533, 4.9967) -> (-8.0889, 9.7803)
  line L102 (-8.0889, 9.7803) -> (-11.2258, 9.7803)
  line L103 (-58.0705, 75.4711) -> (-54.6454, 85.6311)
  line L104 (-54.6454, 85.6311) -> (-52.9822, 85.6311)
  line L105 (-52.9822, 85.6311) -> (-49.5571, 75.4711)
  line L106 (-49.5571, 75.4711) -> (-50.9815, 75.4711)
  line L107 (-50.9815, 75.4711) -> (-51.9037, 78.3116)
  line L108 (-51.9037, 78.3116) -> (-55.7816, 78.3116)
  line L109 (-55.7816, 78.3116) -> (-56.7037, 75.4711)
  line L110 (-56.7037, 75.4711) -> (-58.0705, 75.4711)
  line L111 (-52.2742, 79.4643) -> (-53.8467, 84.2479)
  line L112 (-53.8467, 84.2479) -> (-55.4111, 79.4643)
  line L113 (-55.4111, 79.4643) -> (-52.2742, 79.4643)
  line L114 (-5.4295, 13.7735) -> (-8.8546, 3.6135)
  line L115 (-8.8546, 3.6135) -> (-10.5178, 3.6135)
  line L116 (-10.5178, 3.6135) -> (-13.9429, 13.7735)
  line L117 (-13.9429, 13.7735) -> (-12.5185, 13.7735)
  line L118 (-12.5185, 13.7735) -> (-11.5963, 10.9329)
  line L119 (-11.5963, 10.9329) -> (-7.7184, 10.9329)
  line L120 (-7.7184, 10.9329) -> (-6.7963, 13.7735)
  line L121 (-6.7963, 13.7735) -> (-5.4295, 13.7735)
  line L122 (-11.2258, 9.7803) -> (-9.6533, 4.9967)
  line L123 (-9.6533, 4.9967) -> (-8.0889, 9.7803)
  line L124 (-8.0889, 9.7803) -> (-11.2258, 9.7803)
  point P0 (-31.75, 44.45)
  point P1 (-31.75, 44.45)
  point P2 (-30.7426, 155.7595)
  point P3 (-31.75, 44.4566)
  point P4 (-53.7479, 68.8958)
  point P5 (-53.7479, 68.8958)
  point P6 (-9.7521, 20.0042)
  point P7 (-9.7521, 20.0042)
  point P8 (-19.2735, 44.9329)
  point P9 (-16.6464, 47.093)
  point P10 (-17.0536, 47.558)
  point P11 (-17.8607, 48.3579)
  point P12 (-18.7022, 49.1538)
  point P13 (-19.3099, 49.6753)
  point P14 (-21.7995, 51.3789)
  point P15 (-24.4825, 52.6801)
  point P16 (-27.339, 53.566)
  point P17 (-30.3299, 54.0263)
  point P18 (-31.0576, 54.0671)
  point P19 (-31.8788, 54.0795)
  point P20 (-32.6962, 54.0642)
  point P21 (-33.4164, 54.0207)
  point P22 (-36.5403, 53.5115)
  point P23 (-39.5155, 52.5341)
  point P24 (-42.296, 51.1009)
  point P25 (-44.8432, 49.2346)
  point P26 (-45.3957, 48.7364)
  point P27 (-46.0279, 48.12)
  point P28 (-46.6138, 47.5148)
  point P29 (-46.9896, 47.0797)
  point P30 (-44.3566, 44.9321)
  point P31 (-42.4097, 46.8283)
  point P32 (-40.1768, 48.3986)
  point P33 (-37.7501, 49.5793)
  point P34 (-35.2076, 50.3315)
  point P35 (-33.5322, 50.5864)
  point P36 (-31.8147, 50.6717)
  point P37 (-30.0973, 50.5864)
  point P38 (-28.4217, 50.3315)
  point P39 (-25.8792, 49.5803)
  point P40 (-23.4587, 48.4037)
  point P41 (-21.2339, 46.839)
  point P42 (-23.2452, 41.0656)
  point P43 (-20.6545, 43.2793)
  point P44 (-20.7446, 43.3915)
  point P45 (-20.9905, 43.656)
  point P46 (-21.2887, 43.9679)
  point P47 (-21.6175, 44.3024)
  point P48 (-22.5505, 45.1705)
  point P49 (-23.4975, 45.9121)
  point P50 (-24.5028, 46.5592)
  point P51 (-25.6239, 47.1524)
  point P52 (-26.7382, 47.6281)
  point P53 (-27.9099, 48.0135)
  point P54 (-29.116, 48.3018)
  point P55 (-30.3185, 48.4827)
  point P56 (-30.9625, 48.5251)
  point P57 (-31.8935, 48.5365)
  point P58 (-32.8196, 48.5227)
  point P59 (-33.4163, 48.478)
  point P60 (-35.3346, 48.1205)
  point P61 (-37.1571, 47.5281)
  point P62 (-38.8837, 46.6988)
  point P63 (-40.5311, 45.6279)
  point P64 (-41.0622, 45.1907)
  point P65 (-41.8688, 44.4358)
  point P66 (-42.6526, 43.6661)
  point P67 (-42.977, 43.2779)
  point P68 (-40.3848, 41.0649)
  point P69 (-39.3587, 42.1602)
  point P70 (-38.2302, 43.0936)
  point P71 (-37.0057, 43.8585)
  point P72 (-35.6958, 44.4499)
  point P73 (-32.3299, 45.1442)
  point P74 (-28.9482, 44.7789)
  point P75 (-25.8331, 43.3785)
  point P76 (-27.2128, 37.1424)
  point P77 (-27.1367, 37.051)
  point P78 (-27.071, 36.9831)
  point P79 (-27.0426, 36.9773)
  point P80 (-26.9623, 37.0275)
  point P81 (-25.7875, 38.1305)
  point P82 (-24.5953, 39.2509)
  point P83 (-24.5767, 39.2939)
  point P84 (-24.5825, 39.3115)
  point P85 (-24.6669, 39.4252)
  point P86 (-24.766, 39.5554)
  point P87 (-24.8836, 39.7051)
  point P88 (-25.4949, 40.3815)
  point P89 (-26.2471, 41.0512)
  point P90 (-27.0662, 41.6552)
  point P91 (-27.8611, 42.1187)
  point P92 (-28.3727, 42.3447)
  point P93 (-29.0386, 42.5802)
  point P94 (-29.717, 42.7818)
  point P95 (-30.2747, 42.9036)
  point P96 (-30.7758, 42.9692)
  point P97 (-31.4119, 43.0171)
  point P98 (-32.0314, 43.0416)
  point P99 (-32.4307, 43.0264)
  point P100 (-34.0238, 42.7492)
  point P101 (-35.4689, 42.2479)
  point P102 (-36.776, 41.5149)
  point P103 (-37.9581, 40.5486)
  point P104 (-38.337, 40.1659)
  point P105 (-38.6996, 39.7682)
  point P106 (-39.0151, 39.4003)
  point P107 (-39.0527, 39.2969)
  point P108 (-39.0335, 39.2524)
  point P109 (-37.8444, 38.1327)
  point P110 (-36.672, 37.0301)
  point P111 (-36.5889, 36.978)
  point P112 (-36.5603, 36.9845)
  point P113 (-36.4741, 37.0791)
  point P114 (-36.3741, 37.2003)
  point P115 (-36.2643, 37.3476)
  point P116 (-35.6054, 38.1054)
  point P117 (-34.8084, 38.7362)
  point P118 (-33.9055, 39.2154)
  point P119 (-32.9322, 39.5234)
  point P120 (-32.3612, 39.5988)
  point P121 (-31.6217, 39.6035)
  point P122 (-30.8835, 39.5483)
  point P123 (-30.3165, 39.434)
  point P124 (-29.4512, 39.0947)
  point P125 (-28.6193, 38.5905)
  point P126 (-27.8809, 37.9625)
  point P127 (-27.2937, 37.2545)
  point P128 (-32.3905, 37.4614)
  point P129 (-32.5231, 37.4314)
  point P130 (-33.3556, 37.0457)
  point P131 (-34.0289, 36.4128)
  point P132 (-34.4667, 35.607)
  point P133 (-34.6168, 34.721)
  point P134 (-34.3295, 33.4988)
  point P135 (-33.5302, 32.5168)
  point P136 (-32.3899, 31.9809)
  point P137 (-31.149, 32.0059)
  point P138 (-30.4318, 32.2925)
  point P139 (-29.8377, 32.7398)
  point P140 (-29.3904, 33.3339)
  point P141 (-29.1038, 34.0511)
  point P142 (-29.0802, 35.3061)
  point P143 (-29.6275, 36.4509)
  point P144 (-30.6295, 37.2438)
  point P145 (-31.8739, 37.5142)
  point P146 (-32.0366, 37.5064)
  point P147 (-32.2181, 37.4876)
  point P148 (-10.5703, 22.8165)
  point P149 (-10.4026, 22.4657)
  point P150 (-10.0955, 22.2226)
  point P151 (-9.7141, 22.1398)
  point P152 (-9.6642, 22.1422)
  point P153 (-9.6086, 22.1479)
  point P154 (-9.5557, 22.1559)
  point P155 (-9.5151, 22.1652)
  point P156 (-9.2599, 22.2834)
  point P157 (-9.0536, 22.4773)
  point P158 (-8.9194, 22.7243)
  point P159 (-8.8734, 22.9959)
  point P160 (-8.9615, 23.3705)
  point P161 (-9.2064, 23.6715)
  point P162 (-9.5559, 23.8357)
  point P163 (-9.9363, 23.8281)
  point P164 (-10.1561, 23.7402)
  point P165 (-10.3382, 23.6031)
  point P166 (-10.4753, 23.421)
  point P167 (-10.5631, 23.2012)
  point P168 (-11.1179, 22.2194)
  point P169 (-11.1427, 22.2537)
  point P170 (-11.1661, 22.2818)
  point P171 (-11.1862, 22.3026)
  point P172 (-11.1949, 22.3043)
  point P173 (-11.2195, 22.289)
  point P174 (-11.5796, 21.9509)
  point P175 (-11.945, 21.6075)
  point P176 (-11.9503, 21.5909)
  point P177 (-11.923, 21.5541)
  point P178 (-11.8927, 21.5141)
  point P179 (-11.8566, 21.4683)
  point P180 (-11.6693, 21.2609)
  point P181 (-11.4387, 21.0557)
  point P182 (-11.1876, 20.8705)
  point P183 (-10.944, 20.7285)
  point P184 (-10.7872, 20.6592)
  point P185 (-10.5831, 20.587)
  point P186 (-10.3752, 20.5253)
  point P187 (-10.2042, 20.4879)
  point P188 (-10.0507, 20.4678)
  point P189 (-9.8557, 20.4531)
  point P190 (-9.6658, 20.4456)
  point P191 (-9.5434, 20.4503)
  point P192 (-9.0551, 20.5352)
  point P193 (-8.6122, 20.6889)
  point P194 (-8.2116, 20.9135)
  point P195 (-7.8493, 21.2097)
  point P196 (-7.7331, 21.327)
  point P197 (-7.622, 21.4489)
  point P198 (-7.5253, 21.5617)
  point P199 (-7.5138, 21.5934)
  dimension "d103" = 8.4153
  dimension "d105" = 0.508
  dimension "d106" = 0.508
  dimension "d107" = -2.9972
  dimension "d109" = 9.7536
  dimension "d111" = 2.9972
  dimension "d112" = -2.9972
  constraints: 1088 point on circle, 544 centre point, 138 end point, 2 midpoint, 4 other
  measures "d103" distance of L12.end L14.start
  measures "d105" distance between parallel lines of L15 L7
  measures "d106" distance between parallel lines of L16 L11
  measures "d107" vertical distance of point (-30.743, 155.76) A129.centre
  measures "d109" vertical distance of point (-31.75, 44.457) A265.centre
  measures "d111" vertical distance of point (-53.748, 68.896) A401.centre
  measures "d112" vertical distance of point (-9.752, 20.004) A537.centre
extrude "Extrusion20" add sketch "Sketch17" along normal blind 0.4 contours A167 A166 A165 A164 A163 A162 A161 A160 A159 A158 A157 A156 L40 L39 L38 L37 A155 A154 A153 A152 A151 A150 A149 A148 A147 A146 A145 A144 L36 L35 L34 L33 A143 A142 A141 A140 A139 A138 A137 A136 | A199 A198 A197 A196 A195 A194 A193 A192 A191 A190 A189 A188 A187 A186 A185 A184 L48 L47 L46 L45 A183 A182 A181 A180 A179 A178 A177 A176 L44 L43 L42 L41 A175 A174 A173 A172 A171 A170 A169 A168 | A251 A250 A249 A248 A247 A246 A245 A244 A243 A242 A241 A240 A239 A238 A237 A236 A235 A234 A233 A232 A231 A230 A229 A228 A227 A226 A225 A224 A223 A222 A221 A220 A219 A218 A217 A216 A215 A214 A213 A212 A211 A210 A209 A208 A207 A206 A205 A204 A203 A202 A201 A200 | A271 A270 A269 A268 A267 A266 A265 A264 A263 A262 A261 A260 A259 A258 A257 A256 A255 A254 A253 A252 | A303 A302 A301 A300 A299 A298 A297 A296 A295 A294 A293 A292 L56 L55 L54 L53 A291 A290 A289 A288 A287 A286 A285 A284 A283 A282 A281 A280 L52 L51 L50 L49 A279 A278 A277 A276 A275 A274 A273 A272 | A335 A334 A333 A332 A331 A330 A329 A328 A327 A326 A325 A324 A323 A322 A321 A320 L64 L63 L62 L61 A319 A318 A317 A316 A315 A314 A313 A312 L60 L59 L58 L57 A311 A310 A309 A308 A307 A306 A305 A304 | A387 A386 A385 A384 A383 A382 A381 A380 A379 A378 A377 A376 A375 A374 A373 A372 A371 A370 A369 A368 A367 A366 A365 A364 A363 A362 A361 A360 A359 A358 A357 A356 A355 A354 A353 A352 A351 A350 A349 A348 A347 A346 A345 A344 A343 A342 A341 A340 A339 A338 A337 A336 | A407 A406 A405 A404 A403 A402 A401 A400 A399 A398 A397 A396 A395 A394 A393 A392 A391 A390 A389 A388 | A439 A438 A437 A436 A435 A434 A433 A432 A431 A430 A429 A428 L72 L71 L70 L69 A427 A426 A425 A424 A423 A422 A421 A420 A419 A418 A417 A416 L68 L67 L66 L65 A415 A414 A413 A412 A411 A410 A409 A408 | A471 A470 A469 A468 A467 A466 A465 A464 A463 A462 A461 A460 A459 A458 A457 A456 L80 L79 L78 L77 A455 A454 A453 A452 A451 A450 A449 A448 L76 L75 L74 L73 A447 A446 A445 A444 A443 A442 A441 A440 | A523 A522 A521 A520 A519 A518 A517 A516 A515 A514 A513 A512 A511 A510 A509 A508 A507 A506 A505 A504 A503 A502 A501 A500 A499 A498 A497 A496 A495 A494 A493 A492 A491 A490 A489 A488 A487 A486 A485 A484 A483 A482 A481 A480 A479 A478 A477 A476 A475 A474 A473 A472 | A543 A542 A541 A540 A539 A538 A537 A536 A535 A534 A533 A532 A531 A530 A529 A528 A527 A526 A525 A524 | L81 L82 L83 L84 L85 L86 L87 L88 | L92 L93 L94 L95 L96 L97 L98 L99 bodies 2
sketch "Sketch18" plane through (0, 0, -0.2) normal (0, 0, -1) x (-1, 0, 0)
  line L0 (0, 0) -> (-63.5, 0)
  line L1 (-63.5, 0) -> (-63.5, 88.9)
  line L2 (-63.5, 88.9) -> (0, 88.9)
  line L3 (0, 88.9) -> (0, 0)
  constraints: 8 end point, 2 parallel, 1 horizontal, 1 perpendicular
extrude "Extrusion21" add sketch "Sketch18" along normal blind 0.4 bodies 3
fillet "Fillet2" radius 3.175 8 edges at (63.5, 0, 0.2) (63.5, 88.9, 0.2) (0, 0, 0.2) (0, 88.9, 0.2) (63.5, 0, -0.3) (63.5, 88.9, -0.3) (0, 0, -0.3) (0, 88.9, -0.3)
extrude "Extrusion22" cut sketch "Sketch17" along normal blind 0.4 contours A167 A166 A165 A164 A163 A162 A161 A160 A159 A158 A157 A156 L40 L39 L38 L37 A155 A154 A153 A152 A151 A150 A149 A148 A147 A146 A145 A144 L36 L35 L34 L33 A143 A142 A141 A140 A139 A138 A137 A136 | A199 A198 A197 A196 A195 A194 A193 A192 A191 A190 A189 A188 A187 A186 A185 A184 L48 L47 L46 L45 A183 A182 A181 A180 A179 A178 A177 A176 L44 L43 L42 L41 A175 A174 A173 A172 A171 A170 A169 A168 | A251 A250 A249 A248 A247 A246 A245 A244 A243 A242 A241 A240 A239 A238 A237 A236 A235 A234 A233 A232 A231 A230 A229 A228 A227 A226 A225 A224 A223 A222 A221 A220 A219 A218 A217 A216 A215 A214 A213 A212 A211 A210 A209 A208 A207 A206 A205 A204 A203 A202 A201 A200 | A271 A270 A269 A268 A267 A266 A265 A264 A263 A262 A261 A260 A259 A258 A257 A256 A255 A254 A253 A252 | A303 A302 A301 A300 A299 A298 A297 A296 A295 A294 A293 A292 L56 L55 L54 L53 A291 A290 A289 A288 A287 A286 A285 A284 A283 A282 A281 A280 L52 L51 L50 L49 A279 A278 A277 A276 A275 A274 A273 A272 | A335 A334 A333 A332 A331 A330 A329 A328 A327 A326 A325 A324 A323 A322 A321 A320 L64 L63 L62 L61 A319 A318 A317 A316 A315 A314 A313 A312 L60 L59 L58 L57 A311 A310 A309 A308 A307 A306 A305 A304 | A387 A386 A385 A384 A383 A382 A381 A380 A379 A378 A377 A376 A375 A374 A373 A372 A371 A370 A369 A368 A367 A366 A365 A364 A363 A362 A361 A360 A359 A358 A357 A356 A355 A354 A353 A352 A351 A350 A349 A348 A347 A346 A345 A344 A343 A342 A341 A340 A339 A338 A337 A336 | A407 A406 A405 A404 A403 A402 A401 A400 A399 A398 A397 A396 A395 A394 A393 A392 A391 A390 A389 A388 | A439 A438 A437 A436 A435 A434 A433 A432 A431 A430 A429 A428 L72 L71 L70 L69 A427 A426 A425 A424 A423 A422 A421 A420 A419 A418 A417 A416 L68 L67 L66 L65 A415 A414 A413 A412 A411 A410 A409 A408 | A471 A470 A469 A468 A467 A466 A465 A464 A463 A462 A461 A460 A459 A458 A457 A456 L80 L79 L78 L77 A455 A454 A453 A452 A451 A450 A449 A448 L76 L75 L74 L73 A447 A446 A445 A444 A443 A442 A441 A440 | A523 A522 A521 A520 A519 A518 A517 A516 A515 A514 A513 A512 A511 A510 A509 A508 A507 A506 A505 A504 A503 A502 A501 A500 A499 A498 A497 A496 A495 A494 A493 A492 A491 A490 A489 A488 A487 A486 A485 A484 A483 A482 A481 A480 A479 A478 A477 A476 A475 A474 A473 A472 | A543 A542 A541 A540 A539 A538 A537 A536 A535 A534 A533 A532 A531 A530 A529 A528 A527 A526 A525 A524 | L81 L82 L83 L84 L85 L86 L87 L88 | L92 L93 L94 L95 L96 L97 L98 L99 bodies 3
